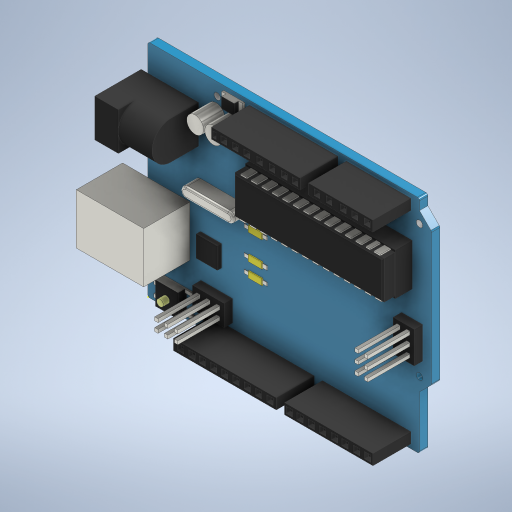
# Autodesk Inventor part: arduino_coloured
Saved by Autodesk Inventor 2024 (Build 280153000, 153)
## iProperties
Created: 2023-06-25
Part Number: arduino_coloured
Material: Generic
Document SubType Name: Modeling
Designer: KETKI GAMRE
Density: 1 g/cm^3
Appearance: Default
Author: KETKI GAMRE
Autodesk Inventor part; units mm, degrees
ref_plane "YZ Plane" through (0, 0, 0) normal (1, 0, 0) x (0, 1, 0)
ref_plane "XZ Plane" through (0, 0, 0) normal (0, 1, 0) x (-1, 0, 0)
ref_plane "XY Plane" through (0, 0, 0) normal (0, 0, 1) x (1, 0, 0)
sketch "Sketch1" plane through (0, 0, 0) normal (0, 0, 1) x (1, 0, 0)
  line L0 (0, 0) -> (0, 52.5)
  line L1 (0, 52.5) -> (64.5, 52.5)
  line L2 (64.5, 52.5) -> (64.5, 50)
  line L3 (64.5, 50) -> (67.3539, 47.1461)
  line L4 (67.3539, 47.1461) -> (67.3539, 15.5601)
  line L5 (67.3539, 15.5601) -> (64.5, 12.7062)
  line L6 (64.5, 12.7062) -> (64.5, 0)
  line L7 (64.5, 0) -> (0, 0)
  dimension "d0" = 52.5
  dimension "d1" = 64.5
  dimension "d2" = 2.5
  dimension "d3" = 4.036
  dimension "d4" = 135
  dimension "d5" = 31.586
  dimension "d6" = 135
  constraints: 16 end point, 4 perpendicular, 2 vertical, 1 parallel, 1 point on line
  measures "d0" distance of L0.start L0.end
  measures "d1" distance of L0.end L1.end
  measures "d2" distance of L1.end L2.end
  measures "d3" distance of L2.end L3.end
  measures "d4" angle of L3 L2
  measures "d5" distance of L3.end L4.end
  measures "d6" angle of L3 L4
extrude "Extrusion1" add sketch "Sketch1" along normal blind 2
fillet "Fillet1" radius 0.5 6 edges at (0, 52.5, 1) (64.5, 52.5, 1) (67.3539, 47.1461, 1) (67.3539, 15.5601, 1) (64.5, 0, 1) (0, 0, 1)
sketch "Sketch2" plane through (0, 0, 2) normal (0, 0, 1) x (1, 0, 0)
  circle A0 centre (64.5, 47.2926) radius 0.75
  circle A1 centre (64.5, 15.9139) radius 0.75
  circle A2 centre (16.5, 49.5) radius 0.75
  circle A3 centre (13.5, 2.5) radius 0.75
  point P0 (0, 0)
  dimension "d11" = 1.5
  dimension "d12" = 1.5
  dimension "d13" = 1.5
  dimension "d14" = 1.5
  constraints: 4 centre point
  measures "d11" diameter of A0
  measures "d12" diameter of A1
  measures "d13" diameter of A2
  measures "d14" diameter of A3
extrude "Extrusion2" cut sketch "Sketch2" against normal blind 2
sketch "Sketch3" plane through (0, 0, 2) normal (0, 0, 1) x (1, 0, 0)
  line L0 (62.438, 51.5) -> (47.138, 51.5)
  line L1 (47.138, 51.5) -> (47.138, 49)
  line L2 (47.138, 49) -> (62.438, 49)
  line L3 (62.438, 49) -> (62.438, 51.5)
  line L4 (45.138, 51.5) -> (24.138, 51.5)
  line L5 (24.138, 51.5) -> (24.138, 49)
  line L6 (24.138, 49) -> (45.138, 49)
  line L7 (45.138, 49) -> (45.138, 51.5)
  point P0 (0, 0)
  dimension "d17" = 15.3
  dimension "d18" = 2.5
  dimension "d19" = 21
  constraints: 16 end point, 4 parallel, 2 horizontal, 2 perpendicular, 2 point on line
  measures "d17" distance of L2.end L1.end
  measures "d18" distance of L1.end L0.end
  measures "d19" distance of L6.end L5.end
extrude "Extrusion3" add sketch "Sketch3" along normal blind 9
sketch "Sketch4" plane through (0, 0, 2) normal (0, 0, 1) x (1, 0, 0)
  circle A0 centre (20.5208, 46.0405) radius 2
  circle A1 centre (16.221, 46.0405) radius 2
  point P0 (0, 0)
  dimension "d22" = 4
  dimension "d23" = 4
  constraints: 2 centre point
  measures "d22" diameter of A0
  measures "d23" diameter of A1
extrude "Extrusion4" add sketch "Sketch4" along normal blind 5
sketch "Sketch5" plane through (0, 0, 2) normal (0, 0, 1) x (1, 0, 0)
  line L0 (23.0063, 51.5) -> (18.0063, 51.5)
  line L1 (18.0063, 51.5) -> (18.0063, 49)
  line L2 (18.0063, 49) -> (23.0063, 49)
  line L3 (23.0063, 49) -> (23.0063, 51.5)
  point P0 (0, 0)
  dimension "d26" = 5
  constraints: 8 end point, 2 parallel, 1 horizontal, 1 perpendicular
  measures "d26" distance of L2.end L1.end
extrude "Extrusion5" add sketch "Sketch5" along normal blind 0.5
sketch "Sketch6" plane through (0, 0, 2.5) normal (0, 0, 1) x (1, 0, 0)
  line L0 (18.0063, 51.5) -> (23.0063, 51.5) projected
  line L1 (18.0063, 49) -> (23.0063, 49) projected
  line L2 (22.006, 51.5) -> (19.006, 51.5)
  line L3 (19.006, 51.5) -> (19.006, 49)
  line L4 (19.006, 49) -> (22.006, 49)
  line L5 (22.006, 49) -> (22.006, 51.5)
  point P0 (0, 0)
  dimension "d29" = 3
  constraints: 8 end point, 2 parallel, 2 point on line, 1 horizontal, 1 perpendicular
  measures "d29" distance of L4.end L3.end
extrude "Extrusion6" add sketch "Sketch6" along normal blind 1
sketch "Sketch7" plane through (0, 0, 2) normal (0, 0, 1) x (1, 0, 0)
  line L0 (62.4512, 1) -> (41.4512, 1)
  line L1 (41.4512, 1) -> (41.4512, 3.5)
  line L2 (41.4512, 3.5) -> (62.4512, 3.5)
  line L3 (62.4512, 3.5) -> (62.4512, 1)
  line L4 (39.4907, 3.5) -> (15.0583, 3.5)
  line L5 (15.0583, 3.5) -> (15.0583, 1)
  line L6 (15.0583, 1) -> (39.4907, 1)
  line L7 (39.4907, 1) -> (39.4907, 3.5)
  point P0 (0, 0)
  dimension "d32" = 21
  dimension "d33" = 2.5
  constraints: 16 end point, 4 parallel, 2 horizontal, 2 perpendicular
  measures "d32" distance of L1.end L2.end
  measures "d33" distance of L0.end L1.end
extrude "Extrusion7" add sketch "Sketch7" along normal blind 9
sketch "Sketch8" plane through (0, 0, 2) normal (0, 0, 1) x (1, 0, 0)
  line L0 (1.8, 1) -> (3.78, 1)
  line L1 (3.78, 1) -> (3.78, 1.8)
  line L2 (3.78, 1.8) -> (1.8, 1.8)
  line L3 (1.8, 1.8) -> (1.8, 1)
  line L4 (1.8, 3.7) -> (3.78, 3.7)
  line L5 (3.78, 3.7) -> (3.78, 4.5)
  line L6 (3.78, 4.5) -> (1.8, 4.5)
  line L7 (1.8, 4.5) -> (1.8, 3.7)
  line L8 (1.8, 5.6) -> (3.78, 5.6)
  line L9 (3.78, 5.6) -> (3.78, 6.4)
  line L10 (3.78, 6.4) -> (1.8, 6.4)
  line L11 (1.8, 6.4) -> (1.8, 5.6)
  line L12 (3.78, 1) -> (9.18, 1)
  line L13 (9.18, 1) -> (9.18, 6.4)
  line L14 (9.18, 6.4) -> (3.78, 6.4)
  line L15 (3.78, 6.4) -> (3.78, 1)
  line L16 (9.18, 6.4) -> (11.16, 6.4)
  line L17 (11.16, 6.4) -> (11.16, 5.6)
  line L18 (11.16, 5.6) -> (9.18, 5.6)
  line L19 (9.18, 5.6) -> (9.18, 6.4)
  line L20 (9.18, 1) -> (11.16, 1)
  line L21 (11.16, 1) -> (11.16, 1.8)
  line L22 (11.16, 1.8) -> (9.18, 1.8)
  line L23 (9.18, 1.8) -> (9.18, 1)
  point P0 (0, 0)
  dimension "d36" = 1.98
  dimension "d37" = 0.8
  dimension "d38" = 0.8
  dimension "d39" = 0.8
  dimension "d40" = 5.4
  dimension "d41" = 1.98
  dimension "d42" = 1.98
  constraints: 48 end point, 12 parallel, 6 horizontal, 6 perpendicular, 2 point on line
  measures "d36" distance of L2.end L1.end
  measures "d37" distance of L1.end L0.end
  measures "d38" distance of L5.end L4.end
  measures "d39" distance of L9.end L8.end
  measures "d40" distance of L14.end L13.end
  measures "d41" distance of L17.end L18.end
  measures "d42" distance of L22.end L21.end
extrude "Extrusion8" add sketch "Sketch8" along normal blind 0.4 contours L3 L2 L1 L0 | L13 L22 L21 L20 | L4 L7 L6 L5 | L13 L16 L17 L18 | L8 L11 L10 L9
sketch "Sketch9" plane through (0, 0, 2) normal (0, 0, 1) x (1, 0, 0)
  line L0 (3.78, 1) -> (3.78, 1.8) projected
  line L1 (11.16, 6.4) -> (9.18, 6.4) projected
  line L2 (3.78, 1) -> (9.18, 1)
  line L3 (9.18, 1) -> (9.18, 6.4)
  line L4 (9.18, 6.4) -> (3.78, 6.4)
  line L5 (3.78, 6.4) -> (3.78, 1)
  point P0 (0, 0)
  constraints: 8 end point, 2 parallel, 1 horizontal, 1 perpendicular
extrude "Extrusion9" add sketch "Sketch9" along normal blind 2
sketch "Sketch10" plane through (0, 0, 4) normal (0, 0, 1) x (1, 0, 0)
  circle A0 centre (6.3835, 3.7) radius 0.785
  point P0 (0, 0)
  dimension "d47" = 1.57
  constraints: 1 centre point
  measures "d47" diameter of A0
extrude "Extrusion10" add sketch "Sketch10" along normal blind 1.5
sketch "Sketch11" plane through (0, 0, 2) normal (0, 0, 1) x (1, 0, 0)
  line L0 (12.606, 4.7021) -> (20.106, 4.7021)
  line L1 (20.106, 4.7021) -> (20.106, 9.7021)
  line L2 (20.106, 9.7021) -> (12.606, 9.7021)
  line L3 (12.606, 9.7021) -> (12.606, 4.7021)
  point P0 (0, 0)
  dimension "d50" = 7.5
  dimension "d51" = 5
  constraints: 8 end point, 2 parallel, 1 horizontal, 1 perpendicular
  measures "d50" distance of L2.end L1.end
  measures "d51" distance of L1.end L0.end
extrude "Extrusion11" add sketch "Sketch11" along normal blind 2
sketch "Sketch12" plane through (0, 0, 4) normal (0, 0, 1) x (1, 0, 0)
  line L0 (13.606, 5.702) -> (14.406, 5.702)
  line L1 (14.406, 5.702) -> (14.406, 6.502)
  line L2 (14.406, 6.502) -> (13.606, 6.502)
  line L3 (13.606, 6.502) -> (13.606, 5.702)
  line L4 (13.606, 7.902) -> (14.406, 7.902)
  line L5 (14.406, 7.902) -> (14.406, 8.702)
  line L6 (14.406, 8.702) -> (13.606, 8.702)
  line L7 (13.606, 8.702) -> (13.606, 7.902)
  line L8 (15.956, 8.702) -> (16.756, 8.702)
  line L9 (16.756, 8.702) -> (16.756, 7.902)
  line L10 (16.756, 7.902) -> (15.956, 7.902)
  line L11 (15.956, 7.902) -> (15.956, 8.702)
  line L12 (15.956, 6.502) -> (16.756, 6.502)
  line L13 (16.756, 6.502) -> (16.756, 5.702)
  line L14 (16.756, 5.702) -> (15.956, 5.702)
  line L15 (15.956, 5.702) -> (15.956, 6.502)
  line L16 (18.306, 8.702) -> (19.106, 8.702)
  line L17 (19.106, 8.702) -> (19.106, 7.902)
  line L18 (19.106, 7.902) -> (18.306, 7.902)
  line L19 (18.306, 7.902) -> (18.306, 8.702)
  line L20 (18.306, 6.502) -> (19.106, 6.502)
  line L21 (19.106, 6.502) -> (19.106, 5.702)
  line L22 (19.106, 5.702) -> (18.306, 5.702)
  line L23 (18.306, 5.702) -> (18.306, 6.502)
  point P0 (0, 0)
  dimension "d54" = 0.8
  dimension "d55" = 0.8
  dimension "d56" = 0.8
  dimension "d57" = 0.8
  dimension "d58" = 0.8
  constraints: 48 end point, 12 parallel, 10 point on line, 6 horizontal, 6 perpendicular
  measures "d54" distance of L2.end L1.end
  measures "d55" distance of L1.end L0.end
  measures "d56" distance of L5.end L4.end
  measures "d57" distance of L9.end L10.end
  measures "d58" distance of L17.end L18.end
extrude "Extrusion12" add sketch "Sketch12" along normal blind 10
sketch "Sketch13" plane through (0, 0, 2) normal (0, 0, 1) x (1, 0, 0)
  line L0 (10, 12.5494) -> (-6, 12.5494)
  line L1 (-6, 12.5494) -> (-6, 24.5494)
  line L2 (-6, 24.5494) -> (10, 24.5494)
  line L3 (10, 24.5494) -> (10, 12.5494)
  point P0 (0, 0)
  dimension "d61" = 16
  dimension "d62" = 12
  constraints: 8 end point, 2 parallel, 1 horizontal, 1 perpendicular
  measures "d61" distance of L1.end L2.end
  measures "d62" distance of L0.end L1.end
extrude "Extrusion13" add sketch "Sketch13" along normal blind 11
sketch "Sketch14" plane through (-6, 12.5494, 2) normal (-1, 0, 0) x (0, 0, 1)
  line L0 (1, 11) -> (8, 11)
  line L1 (10, 9) -> (10, 3)
  line L2 (0, 0) -> (11, 0) projected
  line L3 (1, 1) -> (8, 1)
  line L4 (8, 1) -> (10, 3)
  line L5 (8, 11) -> (10, 9)
  line L6 (1, 11) -> (1, 1)
  point P0 (-2, -12.5494)
  dimension "d65" = 7
  dimension "d66" = 6
  constraints: 12 end point, 3 perpendicular, 2 horizontal
  measures "d65" distance of L0.start L0.end
  measures "d66" distance of L1.start L1.end
extrude "Extrusion14" cut sketch "Sketch14" against normal blind 9
sketch "Sketch15" plane through (3, 12.5494, 2) normal (-1, 0, 0) x (0, 0, 1)
  line L0 (3, 9) -> (6.2, 9)
  line L1 (6.2, 9) -> (6.2, 3)
  line L2 (6.2, 3) -> (3, 3)
  line L3 (3, 3) -> (3, 9)
  point P0 (-2, -12.5494)
  dimension "d69" = 3.2
  dimension "d70" = 6
  constraints: 8 end point, 2 parallel, 1 horizontal, 1 perpendicular
  measures "d69" distance of L1.end L2.end
  measures "d70" distance of L0.end L1.end
extrude "Extrusion15" add sketch "Sketch15" along normal blind 9
sketch "Sketch16" plane through (0, 0, 2) normal (0, 0, 1) x (1, 0, 0)
  line L0 (17.5, 14.702) -> (12.5, 14.702)
  line L1 (12.5, 14.702) -> (12.5, 19.702)
  line L2 (12.5, 19.702) -> (17.5, 19.702)
  line L3 (17.5, 19.702) -> (17.5, 14.702)
  point P0 (0, 0)
  dimension "d73" = 5
  dimension "d74" = 5
  constraints: 8 end point, 2 parallel, 1 horizontal, 1 perpendicular
  measures "d73" distance of L1.end L2.end
  measures "d74" distance of L0.end L1.end
extrude "Extrusion16" add sketch "Sketch16" along normal blind 1
sketch "Sketch17" plane through (0, 0, 2) normal (0, 0, 1) x (1, 0, 0)
  line L0 (24.0339, 16.0009) -> (27.2839, 16.0009)
  line L1 (27.2839, 16.0009) -> (27.2839, 17.5009)
  line L2 (27.2839, 17.5009) -> (24.0339, 17.5009)
  line L3 (24.0339, 17.5009) -> (24.0339, 16.0009)
  line L4 (24.0339, 19.3878) -> (27.2839, 19.3878)
  line L5 (27.2839, 19.3878) -> (27.2839, 20.8878)
  line L6 (27.2839, 20.8878) -> (24.0339, 20.8878)
  line L7 (24.0339, 20.8878) -> (24.0339, 19.3878)
  line L8 (24.0339, 25.4234) -> (27.2839, 25.4234)
  line L9 (27.2839, 25.4234) -> (27.2839, 26.9234)
  line L10 (27.2839, 26.9234) -> (24.0339, 26.9234)
  line L11 (24.0339, 26.9234) -> (24.0339, 25.4234)
  point P0 (0, 0)
  dimension "d77" = 3.25
  dimension "d78" = 1.5
  dimension "d79" = 1.5
  dimension "d80" = 1.5
  constraints: 24 end point, 6 parallel, 4 point on line, 3 horizontal, 3 perpendicular
  measures "d77" distance of L2.end L1.end
  measures "d78" distance of L1.end L0.end
  measures "d79" distance of L5.end L4.end
  measures "d80" distance of L9.end L8.end
extrude "Extrusion17" add sketch "Sketch17" along normal blind 0.2
sketch "Sketch18" plane through (0, 0, 2) normal (0, 0, 1) x (1, 0, 0)
  line L0 (24.0339, 16.0009) -> (24.0339, 17.5009) projected
  line L1 (24.0339, 17.201) -> (22.9339, 17.201)
  line L2 (22.9339, 17.201) -> (22.9339, 16.401)
  line L3 (22.9339, 16.401) -> (24.0339, 16.401)
  line L4 (24.0339, 16.401) -> (24.0339, 17.201)
  line L5 (24.0339, 20.6083) -> (22.9339, 20.6083)
  line L6 (22.9339, 20.6083) -> (22.9339, 19.8083)
  line L7 (22.9339, 19.8083) -> (24.0339, 19.8083)
  line L8 (24.0339, 19.8083) -> (24.0339, 20.6083)
  line L9 (24.0339, 26.6048) -> (22.9339, 26.6048)
  line L10 (22.9339, 26.6048) -> (22.9339, 25.8048)
  line L11 (22.9339, 25.8048) -> (24.0339, 25.8048)
  line L12 (24.0339, 25.8048) -> (24.0339, 26.6048)
  line L13 (27.2839, 17.201) -> (28.3839, 17.201)
  line L14 (28.3839, 17.201) -> (28.3839, 16.401)
  line L15 (28.3839, 16.401) -> (27.2839, 16.401)
  line L16 (27.2839, 16.401) -> (27.2839, 17.201)
  line L17 (27.2839, 20.6083) -> (28.3839, 20.6083)
  line L18 (28.3839, 20.6083) -> (28.3839, 19.6829)
  line L19 (28.3839, 19.6829) -> (27.2839, 19.6829)
  line L20 (27.2839, 19.6829) -> (27.2839, 20.6083)
  line L21 (27.2839, 26.6048) -> (28.3839, 26.6048)
  line L22 (28.3839, 26.6048) -> (28.3839, 25.8048)
  line L23 (28.3839, 25.8048) -> (27.2839, 25.8048)
  line L24 (27.2839, 25.8048) -> (27.2839, 26.6048)
  point P0 (0, 0)
  dimension "d83" = 1.1
  dimension "d84" = 0.8
  dimension "d85" = 0.8
  dimension "d86" = 0.8
  dimension "d87" = 1.1
  constraints: 48 end point, 14 point on line, 12 parallel, 6 horizontal, 6 perpendicular
  measures "d83" distance of L3.end L2.end
  measures "d84" distance of L2.end L1.end
  measures "d85" distance of L6.end L5.end
  measures "d86" distance of L10.end L9.end
  measures "d87" distance of L14.end L15.end
extrude "Extrusion18" add sketch "Sketch18" along normal blind 0.1
sketch "Sketch19" plane through (0, 0, 2) normal (0, 0, 1) x (1, 0, 0)
  line L0 (65.25, 19.4275) -> (60.25, 19.4275)
  line L1 (60.25, 19.4275) -> (60.25, 26.9275)
  line L2 (60.25, 26.9275) -> (65.25, 26.9275)
  line L3 (65.25, 26.9275) -> (65.25, 19.4275)
  point P0 (0, 0)
  dimension "d90" = 5
  dimension "d91" = 7.5
  constraints: 8 end point, 2 parallel, 1 horizontal, 1 perpendicular
  measures "d90" distance of L1.end L2.end
  measures "d91" distance of L0.end L1.end
extrude "Extrusion19" add sketch "Sketch19" along normal blind 2
sketch "Sketch20" plane through (0, 0, 4) normal (0, 0, 1) x (1, 0, 0)
  line L0 (64.25, 25.297) -> (63.45, 25.297)
  line L1 (63.45, 25.297) -> (63.45, 26.097)
  line L2 (63.45, 26.097) -> (64.25, 26.097)
  line L3 (64.25, 26.097) -> (64.25, 25.297)
  line L4 (63.45, 23.747) -> (64.25, 23.747)
  line L5 (64.25, 23.747) -> (64.25, 22.947)
  line L6 (64.25, 22.947) -> (63.45, 22.947)
  line L7 (63.45, 22.947) -> (63.45, 23.747)
  line L8 (63.45, 21.397) -> (64.25, 21.397)
  line L9 (64.25, 21.397) -> (64.25, 20.597)
  line L10 (64.25, 20.597) -> (63.45, 20.597)
  line L11 (63.45, 20.597) -> (63.45, 21.397)
  line L12 (61.95, 26.097) -> (61.15, 26.097)
  line L13 (61.15, 26.097) -> (61.15, 25.297)
  line L14 (61.15, 25.297) -> (61.95, 25.297)
  line L15 (61.95, 25.297) -> (61.95, 26.097)
  line L16 (61.95, 23.747) -> (61.15, 23.747)
  line L17 (61.15, 23.747) -> (61.15, 23.011)
  line L18 (61.15, 23.011) -> (61.95, 23.011)
  line L19 (61.95, 23.011) -> (61.95, 23.747)
  line L20 (61.95, 21.397) -> (61.15, 21.397)
  line L21 (61.15, 21.397) -> (61.15, 20.597)
  line L22 (61.15, 20.597) -> (61.95, 20.597)
  line L23 (61.95, 20.597) -> (61.95, 21.397)
  point P0 (0, 0)
  dimension "d94" = 0.8
  dimension "d95" = 0.8
  dimension "d96" = 0.8
  dimension "d97" = 0.8
  dimension "d98" = 0.8
  constraints: 48 end point, 12 parallel, 10 point on line, 6 horizontal, 6 perpendicular
  measures "d94" distance of L1.end L2.end
  measures "d95" distance of L0.end L1.end
  measures "d96" distance of L4.end L5.end
  measures "d97" distance of L8.end L9.end
  measures "d98" distance of L14.end L13.end
extrude "Extrusion20" add sketch "Sketch20" along normal blind 10
sketch "Sketch21" plane through (0, 0, 2) normal (0, 0, 1) x (1, 0, 0)
  line L0 (62.7549, 33.0002) -> (27.1549, 33.0002)
  line L1 (27.1549, 33.0002) -> (27.1549, 43.0002)
  line L2 (27.1549, 43.0002) -> (62.7549, 43.0002)
  line L3 (62.7549, 43.0002) -> (62.7549, 33.0002)
  point P0 (0, 0)
  dimension "d101" = 35.6
  dimension "d102" = 10
  constraints: 8 end point, 2 parallel, 1 horizontal, 1 perpendicular
  measures "d101" distance of L1.end L2.end
  measures "d102" distance of L0.end L1.end
extrude "Extrusion21" add sketch "Sketch21" along normal blind 4
sketch "Sketch22" plane through (0, 0, 6) normal (0, 0, 1) x (1, 0, 0)
  line L0 (62.655, 42.5) -> (27.255, 42.5)
  line L1 (27.255, 42.5) -> (27.255, 33.5)
  line L2 (27.255, 33.5) -> (62.655, 33.5)
  line L3 (62.655, 33.5) -> (62.655, 42.5)
  point P0 (0, 0)
  dimension "d105" = 35.4
  dimension "d106" = 9
  constraints: 8 end point, 2 parallel, 1 horizontal, 1 perpendicular
  measures "d105" distance of L2.end L1.end
  measures "d106" distance of L1.end L0.end
extrude "Extrusion22" add sketch "Sketch22" along normal blind 2.8
chamfer "Chamfer1" distance 0.283 angle 45 4 edges at (62.655, 38, 8.8) (44.955, 42.5, 8.8) (27.255, 38, 8.8) (44.955, 33.5, 8.8)
sketch "Sketch23" plane through (27.255, 42.5, 6) normal (0, 1, 0) x (1, 0, 0)
  line L0 (0, 0) -> (35.4, 0) projected
  line L1 (34.42, 0) -> (32.92, 0)
  line L2 (32.92, 0) -> (32.92, -2.5)
  line L3 (32.92, -2.5) -> (34.42, -2.5)
  line L4 (34.42, -2.5) -> (34.42, 0)
  line L5 (32.007, 0) -> (31.007, 0)
  line L6 (31.007, 0) -> (31.007, -2.5)
  line L7 (31.007, -2.5) -> (32.007, -2.5)
  line L8 (32.007, -2.5) -> (32.007, 0)
  line L9 (30.027, 0) -> (28.527, 0)
  line L10 (28.527, 0) -> (28.527, -2.5)
  line L11 (28.527, -2.5) -> (30.027, -2.5)
  line L12 (30.027, -2.5) -> (30.027, 0)
  line L13 (27.547, 0) -> (26.047, 0)
  line L14 (26.047, 0) -> (26.047, -2.5)
  line L15 (26.047, -2.5) -> (27.547, -2.5)
  line L16 (27.547, -2.5) -> (27.547, 0)
  line L17 (25.067, 0) -> (23.567, 0)
  line L18 (23.567, 0) -> (23.567, -2.5)
  line L19 (23.567, -2.5) -> (25.067, -2.5)
  line L20 (25.067, -2.5) -> (25.067, 0)
  line L21 (22.587, 0) -> (21.087, 0)
  line L22 (21.087, 0) -> (21.087, -2.5)
  line L23 (21.087, -2.5) -> (22.587, -2.5)
  line L24 (22.587, -2.5) -> (22.587, 0)
  line L25 (20.107, 0) -> (18.607, 0)
  line L26 (18.607, 0) -> (18.607, -2.5)
  line L27 (18.607, -2.5) -> (20.107, -2.5)
  line L28 (20.107, -2.5) -> (20.107, 0)
  line L29 (17.627, 0) -> (16.127, 0)
  line L30 (16.127, 0) -> (16.127, -2.5)
  line L31 (16.127, -2.5) -> (17.627, -2.5)
  line L32 (17.627, -2.5) -> (17.627, 0)
  line L33 (15.147, 0) -> (13.647, 0)
  line L34 (13.647, 0) -> (13.647, -2.5)
  line L35 (13.647, -2.5) -> (15.147, -2.5)
  line L36 (15.147, -2.5) -> (15.147, 0)
  line L37 (35.4999, 0) -> (-0.1001, 0) projected
  line L38 (12.667, 0) -> (11.167, 0)
  line L39 (11.167, 0) -> (11.167, -2.5)
  line L40 (11.167, -2.5) -> (12.667, -2.5)
  line L41 (12.667, -2.5) -> (12.667, 0)
  line L42 (10.187, 0) -> (8.687, 0)
  line L43 (8.687, 0) -> (8.687, -2.5)
  line L44 (8.687, -2.5) -> (10.187, -2.5)
  line L45 (10.187, -2.5) -> (10.187, 0)
  line L46 (7.707, 0) -> (6.207, 0)
  line L47 (6.207, 0) -> (6.207, -2.5)
  line L48 (6.207, -2.5) -> (7.707, -2.5)
  line L49 (7.707, -2.5) -> (7.707, 0)
  line L50 (5.227, 0) -> (3.727, 0)
  line L51 (3.727, 0) -> (3.727, -2.5)
  line L52 (3.727, -2.5) -> (5.227, -2.5)
  line L53 (5.227, -2.5) -> (5.227, 0)
  line L54 (2.747, 0) -> (1.247, 0)
  line L55 (1.247, 0) -> (1.247, -2.5)
  line L56 (1.247, -2.5) -> (2.747, -2.5)
  line L57 (2.747, -2.5) -> (2.747, 0)
  point P0 (-27.255, 6)
  point P1 (32.007, 0)
  point P2 (30.027, 0)
  point P3 (27.547, 0)
  point P4 (26.047, 0)
  point P5 (23.567, 0)
  point P6 (21.087, 0)
  point P7 (18.607, 0)
  point P8 (17.627, 0)
  point P9 (16.127, 0)
  point P10 (15.147, 0)
  point P11 (8.687, 0)
  point P12 (7.707, 0)
  point P13 (6.207, 0)
  point P14 (5.227, 0)
  point P15 (2.747, 0)
  point P16 (1.247, 0)
  dimension "d112" = 1.5
  dimension "d113" = 2.5
  dimension "d114" = 1
  dimension "d115" = 1.5
  dimension "d116" = 2.5
  dimension "d117" = 1.5
  dimension "d118" = 2.5
  dimension "d119" = 1.5
  dimension "d120" = 2.5
  dimension "d121" = 1.5
  dimension "d122" = 2.5
  dimension "d123" = 1.5
  dimension "d124" = 2.5
  dimension "d125" = 1.5
  dimension "d126" = 2.5
  dimension "d127" = 1.5
  dimension "d128" = 2.5
  dimension "d129" = 1.5
  dimension "d130" = 2.5
  dimension "d131" = 1.5
  dimension "d132" = 2.5
  dimension "d133" = 1.5
  dimension "d134" = 2.5
  dimension "d135" = 1.5
  dimension "d136" = 2.5
  dimension "d137" = 1.5
  dimension "d138" = 2.5
  constraints: 112 end point, 28 parallel, 14 horizontal, 14 perpendicular, 10 point on line, 5 other
  measures "d112" distance of L3.end L2.end
  measures "d113" distance of L2.end L1.end
  measures "d114" distance of L7.end L6.end
  measures "d115" distance of L11.end L10.end
  measures "d116" distance of L10.end L9.end
  measures "d117" distance of L15.end L14.end
  measures "d118" distance of L14.end L13.end
  measures "d119" distance of L19.end L18.end
  measures "d120" distance of L18.end L17.end
  measures "d121" distance of L23.end L22.end
  measures "d122" distance of L22.end L21.end
  measures "d123" distance of L27.end L26.end
  measures "d124" distance of L26.end L25.end
  measures "d125" distance of L31.end L30.end
  measures "d126" distance of L30.end L29.end
  measures "d127" distance of L35.end L34.end
  measures "d128" distance of L34.end L33.end
  measures "d129" distance of L40.end L39.end
  measures "d130" distance of L39.end L38.end
  measures "d131" distance of L44.end L43.end
  measures "d132" distance of L43.end L42.end
  measures "d133" distance of L48.end L47.end
  measures "d134" distance of L47.end L46.end
  measures "d135" distance of L52.end L51.end
  measures "d136" distance of L51.end L50.end
  measures "d137" distance of L56.end L55.end
  measures "d138" distance of L55.end L54.end
extrude "Extrusion23" add sketch "Sketch23" along normal blind 0.3
sketch "Sketch24" plane through (27.255, 33.5, 6) normal (0, -1, 0) x (1, 0, 0)
  line L0 (35.4, 0) -> (0, 0) projected
  line L1 (0.98, 0) -> (2.48, 0)
  line L2 (2.48, 0) -> (2.48, 2.5)
  line L3 (2.48, 2.5) -> (0.98, 2.5)
  line L4 (0.98, 2.5) -> (0.98, 0)
  line L5 (3.46, 0) -> (4.96, 0)
  line L6 (4.96, 0) -> (4.96, 2.5)
  line L7 (4.96, 2.5) -> (3.46, 2.5)
  line L8 (3.46, 2.5) -> (3.46, 0)
  line L9 (5.94, 0) -> (7.44, 0)
  line L10 (7.44, 0) -> (7.44, 2.5)
  line L11 (7.44, 2.5) -> (5.94, 2.5)
  line L12 (5.94, 2.5) -> (5.94, 0)
  line L13 (8.42, 0) -> (9.92, 0)
  line L14 (9.92, 0) -> (9.92, 2.5)
  line L15 (9.92, 2.5) -> (8.42, 2.5)
  line L16 (8.42, 2.5) -> (8.42, 0)
  line L17 (10.9, 0) -> (12.4, 0)
  line L18 (12.4, 0) -> (12.4, 2.5)
  line L19 (12.4, 2.5) -> (10.9, 2.5)
  line L20 (10.9, 2.5) -> (10.9, 0)
  line L21 (13.38, 0) -> (14.88, 0)
  line L22 (14.88, 0) -> (14.88, 2.5)
  line L23 (14.88, 2.5) -> (13.38, 2.5)
  line L24 (13.38, 2.5) -> (13.38, 0)
  line L25 (15.86, 0) -> (17.36, 0)
  line L26 (17.36, 0) -> (17.36, 2.5)
  line L27 (17.36, 2.5) -> (15.86, 2.5)
  line L28 (15.86, 2.5) -> (15.86, 0)
  line L29 (-0.1001, 0) -> (35.4999, 0) projected
  line L30 (18.34, 0) -> (19.84, 0)
  line L31 (19.84, 0) -> (19.84, 2.5)
  line L32 (19.84, 2.5) -> (18.34, 2.5)
  line L33 (18.34, 2.5) -> (18.34, 0)
  line L34 (20.82, 0) -> (22.32, 0)
  line L35 (22.32, 0) -> (22.32, 2.5)
  line L36 (22.32, 2.5) -> (20.82, 2.5)
  line L37 (20.82, 2.5) -> (20.82, 0)
  line L38 (23.3, 0) -> (24.8, 0)
  line L39 (24.8, 0) -> (24.8, 2.5)
  line L40 (24.8, 2.5) -> (23.3, 2.5)
  line L41 (23.3, 2.5) -> (23.3, 0)
  line L42 (25.78, 0) -> (27.28, 0)
  line L43 (27.28, 0) -> (27.28, 2.5)
  line L44 (27.28, 2.5) -> (25.78, 2.5)
  line L45 (25.78, 2.5) -> (25.78, 0)
  line L46 (28.26, 0) -> (29.76, 0)
  line L47 (29.76, 0) -> (29.76, 2.5)
  line L48 (29.76, 2.5) -> (28.26, 2.5)
  line L49 (28.26, 2.5) -> (28.26, 0)
  line L50 (30.74, 0) -> (32.24, 0)
  line L51 (32.24, 0) -> (32.24, 2.5)
  line L52 (32.24, 2.5) -> (30.74, 2.5)
  line L53 (30.74, 2.5) -> (30.74, 0)
  line L54 (33.22, 0) -> (34.72, 0)
  line L55 (34.72, 0) -> (34.72, 2.5)
  line L56 (34.72, 2.5) -> (33.22, 2.5)
  line L57 (33.22, 2.5) -> (33.22, 0)
  point P0 (-27.255, -6)
  point P1 (2.48, 0)
  point P2 (3.46, 0)
  point P3 (4.96, 0)
  point P4 (5.94, 0)
  point P5 (7.44, 0)
  point P6 (9.92, 0)
  point P7 (10.9, 0)
  point P8 (14.88, 0)
  point P9 (15.86, 0)
  point P10 (17.36, 0)
  point P11 (18.34, 0)
  point P12 (20.82, 0)
  point P13 (22.32, 0)
  point P14 (24.8, 0)
  point P15 (27.28, 0)
  point P16 (29.76, 0)
  point P17 (32.24, 0)
  dimension "d141" = 1.5
  dimension "d142" = 2.5
  dimension "d143" = 1.5
  dimension "d144" = 2.5
  dimension "d145" = 1.5
  dimension "d146" = 2.5
  dimension "d147" = 1.5
  dimension "d148" = 2.5
  dimension "d149" = 1.5
  dimension "d150" = 2.5
  dimension "d151" = 1.5
  dimension "d152" = 2.5
  dimension "d153" = 1.5
  dimension "d154" = 2.5
  dimension "d155" = 1.5
  dimension "d156" = 2.5
  dimension "d157" = 1.5
  dimension "d158" = 2.5
  dimension "d159" = 1.5
  dimension "d160" = 2.5
  dimension "d161" = 1.5
  dimension "d162" = 2.5
  dimension "d163" = 1.5
  dimension "d164" = 2.5
  dimension "d165" = 1.5
  dimension "d166" = 2.5
  dimension "d167" = 1.5
  constraints: 112 end point, 28 parallel, 14 horizontal, 14 perpendicular, 12 point on line, 5 other
  measures "d141" distance of L3.end L2.end
  measures "d142" distance of L2.end L1.end
  measures "d143" distance of L7.end L6.end
  measures "d144" distance of L6.end L5.end
  measures "d145" distance of L11.end L10.end
  measures "d146" distance of L10.end L9.end
  measures "d147" distance of L15.end L14.end
  measures "d148" distance of L14.end L13.end
  measures "d149" distance of L19.end L18.end
  measures "d150" distance of L18.end L17.end
  measures "d151" distance of L23.end L22.end
  measures "d152" distance of L22.end L21.end
  measures "d153" distance of L27.end L26.end
  measures "d154" distance of L26.end L25.end
  measures "d155" distance of L32.end L31.end
  measures "d156" distance of L31.end L30.end
  measures "d157" distance of L36.end L35.end
  measures "d158" distance of L35.end L34.end
  measures "d159" distance of L40.end L39.end
  measures "d160" distance of L39.end L38.end
  measures "d161" distance of L44.end L43.end
  measures "d162" distance of L43.end L42.end
  measures "d163" distance of L48.end L47.end
  measures "d164" distance of L47.end L46.end
  measures "d165" distance of L52.end L51.end
  measures "d166" distance of L51.end L50.end
  measures "d167" distance of L56.end L55.end
extrude "Extrusion24" add sketch "Sketch24" along normal blind 0.3
sketch "Sketch25" plane through (0, 0, 2) normal (0, 0, 1) x (1, 0, 0)
  line L0 (12.5, 28.0885) -> (22.5, 28.0885)
  line L1 (22.5, 30.5885) -> (12.5, 30.5885)
  arc A0 (12.5, 30.5885) -> (12.5, 28.0885) centre (12.5, 29.3385) ccw
  arc A1 (22.5, 28.0885) -> (22.5, 30.5885) centre (22.5, 29.3385) ccw
  point P0 (0, 0)
  dimension "d171" = 2.5
  dimension "d172" = 2.5
  dimension "d173" = 2.5
  constraints: 4 end point, 4 point on circle, 2 centre point, 1 horizontal
  measures "d171" distance of L0.end L1.start
  measures "d172" diameter of A0
  measures "d173" diameter of A1
extrude "Extrusion25" add sketch "Sketch25" along normal blind 3.5
fillet "Fillet2" radius 0.5 4 edges at (23.75, 29.3385, 5.5) (17.5, 30.5885, 5.5) (11.25, 29.3385, 5.5) (17.5, 28.0885, 5.5)
sketch "Sketch26" plane through (0, 0, 11) normal (0, 0, 1) x (1, 0, 0)
  line L0 (61.7734, 49.5928) -> (60.3734, 49.5928)
  line L1 (60.3734, 49.5928) -> (60.3734, 50.9848)
  line L2 (60.3734, 50.9848) -> (61.7734, 50.9848)
  line L3 (61.7734, 50.9848) -> (61.7734, 49.5928)
  line L4 (58.8501, 49.5928) -> (57.4501, 49.5928)
  line L5 (57.4501, 49.5928) -> (57.4501, 50.9928)
  line L6 (57.4501, 50.9928) -> (58.8501, 50.9928)
  line L7 (58.8501, 50.9928) -> (58.8501, 49.5928)
  line L8 (56.0659, 49.5928) -> (54.6659, 49.5928)
  line L9 (54.6659, 49.5928) -> (54.6659, 50.9928)
  line L10 (54.6659, 50.9928) -> (56.0659, 50.9928)
  line L11 (56.0659, 50.9928) -> (56.0659, 49.5928)
  line L12 (52.7249, 49.5928) -> (51.3249, 49.5928)
  line L13 (51.3249, 49.5928) -> (51.3249, 50.9928)
  line L14 (51.3249, 50.9928) -> (52.7249, 50.9928)
  line L15 (52.7249, 50.9928) -> (52.7249, 49.5928)
  line L16 (49.8712, 50.9928) -> (48.4712, 50.9928)
  line L17 (48.4712, 50.9928) -> (48.4712, 49.5928)
  line L18 (48.4712, 49.5928) -> (49.8712, 49.5928)
  line L19 (49.8712, 49.5928) -> (49.8712, 50.9928)
  point P0 (0, 0)
  dimension "d177" = 1.4
  dimension "d178" = 1.4
  dimension "d179" = 1.4
  dimension "d180" = 1.4
  dimension "d181" = 1.4
  dimension "d182" = 1.4
  dimension "d183" = 1.4
  dimension "d184" = 1.4
  dimension "d185" = 1.4
  constraints: 40 end point, 10 parallel, 5 horizontal, 5 perpendicular, 2 point on line
  measures "d177" distance of L1.end L2.end
  measures "d178" distance of L5.end L6.end
  measures "d179" distance of L4.end L5.end
  measures "d180" distance of L9.end L10.end
  measures "d181" distance of L8.end L9.end
  measures "d182" distance of L13.end L14.end
  measures "d183" distance of L12.end L13.end
  measures "d184" distance of L18.end L17.end
  measures "d185" distance of L17.end L16.end
extrude "Extrusion26" cut sketch "Sketch26" against normal blind 1
sketch "Sketch27" plane through (0, 0, 11) normal (0, 0, 1) x (1, 0, 0)
  line L0 (44.6514, 49.4703) -> (43.2514, 49.4703)
  line L1 (43.2514, 49.4703) -> (43.2514, 50.8703)
  line L2 (43.2514, 50.8703) -> (44.6514, 50.8703)
  line L3 (44.6514, 50.8703) -> (44.6514, 49.4703)
  line L4 (42.0706, 49.4703) -> (40.6706, 49.4703)
  line L5 (40.6706, 49.4703) -> (40.6706, 50.8703)
  line L6 (40.6706, 50.8703) -> (42.0706, 50.8703)
  line L7 (42.0706, 50.8703) -> (42.0706, 49.4703)
  line L8 (39.177, 50.8703) -> (37.777, 50.8703)
  line L9 (37.777, 50.8703) -> (37.777, 49.4703)
  line L10 (37.777, 49.4703) -> (39.177, 49.4703)
  line L11 (39.177, 49.4703) -> (39.177, 50.8703)
  line L12 (36.2443, 49.4703) -> (34.8443, 49.4703)
  line L13 (34.8443, 49.4703) -> (34.8443, 50.8703)
  line L14 (34.8443, 50.8703) -> (36.2443, 50.8703)
  line L15 (36.2443, 50.8703) -> (36.2443, 49.4703)
  line L16 (33.1943, 50.8703) -> (31.7943, 50.8703)
  line L17 (31.7943, 50.8703) -> (31.7943, 49.4703)
  line L18 (31.7943, 49.4703) -> (33.1943, 49.4703)
  line L19 (33.1943, 49.4703) -> (33.1943, 50.8703)
  line L20 (30.4571, 49.4703) -> (29.0571, 49.4703)
  line L21 (29.0571, 49.4703) -> (29.0571, 50.8703)
  line L22 (29.0571, 50.8703) -> (30.4571, 50.8703)
  line L23 (30.4571, 50.8703) -> (30.4571, 49.4703)
  line L24 (27.7199, 50.8703) -> (26.3199, 50.8703)
  line L25 (26.3199, 50.8703) -> (26.3199, 49.4703)
  line L26 (26.3199, 49.4703) -> (27.7199, 49.4703)
  line L27 (27.7199, 49.4703) -> (27.7199, 50.8703)
  line L28 (25.2565, 49.4703) -> (24.3962, 49.4703)
  line L29 (24.3962, 49.4703) -> (24.3962, 50.8703)
  line L30 (24.3962, 50.8703) -> (25.2565, 50.8703)
  line L31 (25.2565, 50.8703) -> (25.2565, 49.4703)
  point P0 (0, 0)
  dimension "d188" = 1.4
  dimension "d189" = 1.4
  dimension "d190" = 1.4
  dimension "d191" = 1.4
  dimension "d192" = 1.4
  dimension "d193" = 1.4
  dimension "d194" = 1.4
  dimension "d195" = 1.4
  constraints: 64 end point, 16 parallel, 13 point on line, 8 horizontal, 8 perpendicular
  measures "d188" distance of L1.end L2.end
  measures "d189" distance of L0.end L1.end
  measures "d190" distance of L5.end L6.end
  measures "d191" distance of L10.end L9.end
  measures "d192" distance of L13.end L14.end
  measures "d193" distance of L18.end L17.end
  measures "d194" distance of L21.end L22.end
  measures "d195" distance of L26.end L25.end
extrude "Extrusion27" cut sketch "Sketch27" against normal blind 1
sketch "Sketch28" plane through (0, 0, 11) normal (0, 0, 1) x (1, 0, 0)
  line L0 (61.9446, 1.4316) -> (60.4446, 1.4316)
  line L1 (60.4446, 1.4316) -> (60.4446, 2.9316)
  line L2 (60.4446, 2.9316) -> (61.9446, 2.9316)
  line L3 (61.9446, 2.9316) -> (61.9446, 1.4316)
  line L4 (59.301, 2.9316) -> (57.801, 2.9316)
  line L5 (57.801, 2.9316) -> (57.801, 1.4316)
  line L6 (57.801, 1.4316) -> (59.301, 1.4316)
  line L7 (59.301, 1.4316) -> (59.301, 2.9316)
  line L8 (56.5839, 1.4316) -> (55.0839, 1.4316)
  line L9 (55.0839, 1.4316) -> (55.0839, 2.9316)
  line L10 (55.0839, 2.9316) -> (56.5839, 2.9316)
  line L11 (56.5839, 2.9316) -> (56.5839, 1.4316)
  line L12 (54.0872, 2.9316) -> (52.5872, 2.9316)
  line L13 (52.5872, 2.9316) -> (52.5872, 1.4316)
  line L14 (52.5872, 1.4316) -> (54.0872, 1.4316)
  line L15 (54.0872, 1.4316) -> (54.0872, 2.9316)
  line L16 (51.2967, 1.4316) -> (49.7967, 1.4316)
  line L17 (49.7967, 1.4316) -> (49.7967, 2.9316)
  line L18 (49.7967, 2.9316) -> (51.2967, 2.9316)
  line L19 (51.2967, 2.9316) -> (51.2967, 1.4316)
  line L20 (48.5429, 2.9316) -> (47.0429, 2.9316)
  line L21 (47.0429, 2.9316) -> (47.0429, 1.4316)
  line L22 (47.0429, 1.4316) -> (48.5429, 1.4316)
  line L23 (48.5429, 1.4316) -> (48.5429, 2.9316)
  line L24 (45.8625, 1.4316) -> (44.3625, 1.4316)
  line L25 (44.3625, 1.4316) -> (44.3625, 2.9316)
  line L26 (44.3625, 2.9316) -> (45.8625, 2.9316)
  line L27 (45.8625, 2.9316) -> (45.8625, 1.4316)
  line L28 (43.3291, 2.9316) -> (41.8291, 2.9316)
  line L29 (41.8291, 2.9316) -> (41.8291, 1.4316)
  line L30 (41.8291, 1.4316) -> (43.3291, 1.4316)
  line L31 (43.3291, 1.4316) -> (43.3291, 2.9316)
  point P0 (0, 0)
  dimension "d198" = 1.5
  dimension "d199" = 1.5
  dimension "d200" = 1.5
  dimension "d201" = 1.5
  dimension "d202" = 1.5
  dimension "d203" = 1.5
  dimension "d204" = 1.5
  dimension "d205" = 1.5
  dimension "d206" = 1.5
  constraints: 64 end point, 16 parallel, 14 point on line, 8 horizontal, 8 perpendicular
  measures "d198" distance of L1.end L2.end
  measures "d199" distance of L0.end L1.end
  measures "d200" distance of L6.end L5.end
  measures "d201" distance of L9.end L10.end
  measures "d202" distance of L14.end L13.end
  measures "d203" distance of L17.end L18.end
  measures "d204" distance of L22.end L21.end
  measures "d205" distance of L25.end L26.end
  measures "d206" distance of L30.end L29.end
extrude "Extrusion28" cut sketch "Sketch28" against normal blind 1
sketch "Sketch29" plane through (0, 0, 11) normal (0, 0, 1) x (1, 0, 0)
  line L0 (38.7414, 1.5074) -> (37.2414, 1.5074)
  line L1 (37.2414, 1.5074) -> (37.2414, 3.0074)
  line L2 (37.2414, 3.0074) -> (38.7414, 3.0074)
  line L3 (38.7414, 3.0074) -> (38.7414, 1.5074)
  line L4 (36.021, 3.0074) -> (34.521, 3.0074)
  line L5 (34.521, 3.0074) -> (34.521, 1.5074)
  line L6 (34.521, 1.5074) -> (36.021, 1.5074)
  line L7 (36.021, 1.5074) -> (36.021, 3.0074)
  line L8 (33.3368, 1.5074) -> (31.8368, 1.5074)
  line L9 (31.8368, 1.5074) -> (31.8368, 3.0074)
  line L10 (31.8368, 3.0074) -> (33.3368, 3.0074)
  line L11 (33.3368, 3.0074) -> (33.3368, 1.5074)
  line L12 (30.6889, 3.0074) -> (29.1889, 3.0074)
  line L13 (29.1889, 3.0074) -> (29.1889, 1.5074)
  line L14 (29.1889, 1.5074) -> (30.6889, 1.5074)
  line L15 (30.6889, 1.5074) -> (30.6889, 3.0074)
  line L16 (28.0047, 1.5074) -> (26.5047, 1.5074)
  line L17 (26.5047, 1.5074) -> (26.5047, 3.0074)
  line L18 (26.5047, 3.0074) -> (28.0047, 3.0074)
  line L19 (28.0047, 3.0074) -> (28.0047, 1.5074)
  line L20 (25.3567, 3.0074) -> (23.8567, 3.0074)
  line L21 (23.8567, 3.0074) -> (23.8567, 1.5074)
  line L22 (23.8567, 1.5074) -> (25.3567, 1.5074)
  line L23 (25.3567, 1.5074) -> (25.3567, 3.0074)
  line L24 (22.7088, 1.5074) -> (21.2088, 1.5074)
  line L25 (21.2088, 1.5074) -> (21.2088, 3.0074)
  line L26 (21.2088, 3.0074) -> (22.7088, 3.0074)
  line L27 (22.7088, 3.0074) -> (22.7088, 1.5074)
  line L28 (20.206, 3.0074) -> (18.706, 3.0074)
  line L29 (18.706, 3.0074) -> (18.706, 1.5074)
  line L30 (18.706, 1.5074) -> (20.206, 1.5074)
  line L31 (20.206, 1.5074) -> (20.206, 3.0074)
  line L32 (17.5581, 1.5074) -> (16.0581, 1.5074)
  line L33 (16.0581, 1.5074) -> (16.0581, 3.0074)
  line L34 (16.0581, 3.0074) -> (17.5581, 3.0074)
  line L35 (17.5581, 3.0074) -> (17.5581, 1.5074)
  point P0 (0, 0)
  dimension "d209" = 1.5
  dimension "d210" = 1.5
  dimension "d211" = 1.5
  dimension "d212" = 1.5
  dimension "d213" = 1.5
  dimension "d214" = 1.5
  dimension "d215" = 1.5
  dimension "d216" = 1.5
  dimension "d217" = 1.5
  dimension "d218" = 1.5
  constraints: 72 end point, 18 parallel, 16 point on line, 9 horizontal, 9 perpendicular
  measures "d209" distance of L1.end L2.end
  measures "d210" distance of L0.end L1.end
  measures "d211" distance of L6.end L5.end
  measures "d212" distance of L9.end L10.end
  measures "d213" distance of L14.end L13.end
  measures "d214" distance of L17.end L18.end
  measures "d215" distance of L22.end L21.end
  measures "d216" distance of L25.end L26.end
  measures "d217" distance of L30.end L29.end
  measures "d218" distance of L33.end L34.end
extrude "Extrusion29" cut sketch "Sketch29" against normal blind 1
sketch "Sketch30" plane through (0, 0, 2) normal (0, 0, 1) x (1, 0, 0)
  point P0 (0, 0)
sketch "Sketch31" plane through (0, 0, 2) normal (0, 0, 1) x (1, 0, 0)
  line L0 (4, 37) -> (-1.6, 37)
  line L1 (-1.6, 37) -> (-1.6, 46)
  line L2 (-1.6, 46) -> (4, 46)
  line L3 (4, 46) -> (4, 37)
  point P0 (0, 0)
  dimension "d221" = 5.6
  dimension "d222" = 9
  constraints: 8 end point, 2 parallel, 1 horizontal, 1 perpendicular
  measures "d221" distance of L1.end L2.end
  measures "d222" distance of L0.end L1.end
extrude "Extrusion30" add sketch "Sketch31" along normal blind 11
sketch "Sketch32" plane through (0, 0, 2) normal (0, 0, 1) x (1, 0, 0)
  line L0 (4, 46) -> (4, 37) projected
  line L1 (4, 46) -> (12, 46)
  line L2 (12, 46) -> (12, 37)
  line L3 (12, 37) -> (4, 37)
  line L4 (4, 37) -> (4, 46)
  point P0 (0, 0)
  dimension "d225" = 8
  constraints: 8 end point, 2 parallel, 1 horizontal, 1 perpendicular
  measures "d225" distance of L2.end L3.end
extrude "Extrusion31" add sketch "Sketch32" along normal blind 6.5
sketch "Sketch33" plane through (4, 37, 13) normal (1, 0, 0) x (0, 0, -1)
  line L0 (4.5, 0) -> (4.5, 9) projected
  circle A0 centre (4.5, 4.5) radius 4.5
  line L1 (4.5, 9) -> (0, 9) projected
  point P0 (13, -37)
  constraints: 1 centre point, 1 midpoint, 1 tangent
extrude "Extrusion32" add sketch "Sketch33" along normal blind 8 contours A0 L0 picked at (3.0109, 4.6808)
sketch "Sketch34" plane through (-1.6, 37, 2) normal (-1, 0, 0) x (0, 0, 1)
  circle A0 centre (6.5, 4.5) radius 3
  point P0 (-2, -37)
  dimension "d230" = 6
  constraints: 1 centre point
  measures "d230" diameter of A0
extrude "Extrusion33" cut sketch "Sketch34" against normal blind 8
sketch "Sketch35" plane through (6.4, 41.5, 8.5) normal (-1, 0, 0) x (0, 0, 1)
  circle A0 centre (0, 0) radius 0.6
  point P0 (-8.5, -41.5)
  dimension "d233" = 1.2
  constraints: 1 centre point
  measures "d233" diameter of A0
extrude "Extrusion34" add sketch "Sketch35" along normal blind 8
body "Solid1"
